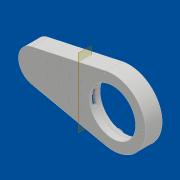
# Autodesk Inventor part: 101-bottom
Saved by Autodesk Inventor 2018 (Build 220112000, 112)
## iProperties
Created: 2019-11-07
Part Number: 101-bottom
Material: Generic
Document SubType Name: Modeling
Designer: Bunny320
Density: 1 g/cm^3
Appearance: Default
Author: Bunny320
Autodesk Inventor part; units mm, degrees
ref_plane "XZ Plane" through (0, 0, 0) normal (0, 1, 0) x (-1, 0, 0)
ref_plane "XY Plane" through (0, 0, 0) normal (0, 0, 1) x (1, 0, 0)
sketch "Sketch2" plane through (0, 0, 0) normal (0, 1, 0) x (-1, 0, 0)
  circle A0 centre (0, 0) radius 27.5
  circle A1 centre (-141.8, 0) radius 57.5
  line L0 (5.8181, -26.8775) -> (-129.635, -56.1984)
  line L1 (5.8181, 26.8775) -> (-129.635, 56.1984)
  dimension "d5" = 141.8
  dimension "d6" = 55
  dimension "d7" = 115
  constraints: 4 end point, 4 point on circle, 4 tangent, 2 centre point, 1 coincident, 1 horizontal alignment
  measures "d5" distance of A1.centre point (0, 0)
  measures "d6" diameter of A0
  measures "d7" diameter of A1
extrude "Extrusion2" add sketch "Sketch2" along normal blind 4
sketch "Sketch5" plane through (0, 4, 0) normal (0, 1, 0) x (1, 0, 0)
  arc A0 (129.635, -56.1984) -> (129.635, 56.1984) centre (141.8, 0) ccw projected
  circle A1 centre (141.8, 0) radius 45
  circle A2 centre (141.8, 0) radius 48
  point P0 (0, 0)
  dimension "d17" = 90
  dimension "d18" = 96
  constraints: 2 centre point, 2 coincident
  measures "d17" diameter of A1
  measures "d18" diameter of A2
extrude "Extrusion5" add sketch "Sketch5" along normal blind 18
sketch "Sketch6" plane through (141.8, 4, 0) normal (0, 1, 0) x (1, 0, 0)
  arc A0 (-12.165, -56.1984) -> (-12.165, 56.1984) centre (0, 0) ccw projected
  circle A1 centre (0, 0) radius 42
  point P0 (-141.8, 0)
  dimension "d21" = 84
  constraints: 1 centre point, 1 coincident
  measures "d21" diameter of A1
extrude "Extrusion6" cut sketch "Sketch6" against normal through all
sketch "Sketch9" plane through (0, 4, 0) normal (0, 1, 0) x (1, 0, 0)
  line L0 (-5.5, -9) -> (5.5, -9) construction
  line L1 (5.5, -9) -> (5.5, 9) construction
  line L2 (5.5, 9) -> (-5.5, 9) construction
  line L3 (-5.5, 9) -> (-5.5, -9) construction
  line L4 (-5.5, -9) -> (5.5, 9) construction
  line L5 (5.5, -9) -> (-5.5, 9) construction
  circle A0 centre (5.5, 9) radius 3
  circle A1 centre (-5.5, 9) radius 3
  circle A2 centre (-5.5, -9) radius 3
  circle A3 centre (5.5, -9) radius 3
  point P0 (0, 0)
  dimension "d33" = 11
  dimension "d34" = 18
  dimension "d35" = 6
  constraints: 12 end point, 4 centre point, 4 coincident, 3 equal radius, 2 midpoint, 2 parallel, 1 horizontal, 1 perpendicular
  measures "d33" distance of L1.end L2.end
  measures "d34" distance of L2.end L0.start
  measures "d35" diameter of A1
extrude "Extrusion7" add sketch "Sketch9" along normal blind 9.75
sketch "Sketch10" plane through (5.5, 13.75, -9) normal (0, 1, 0) x (1, 0, 0)
  circle A0 centre (-11, 0) radius 3 projected
  circle A1 centre (-11, -18) radius 3 projected
  circle A2 centre (0, -18) radius 3 projected
  circle A3 centre (0, 0) radius 3 projected
  point P0 (-5.5, -9)
  constraints: 4 coincident
hole "Hole2" at (-5.5, 13.75, -9) at (-5.5, 13.75, 9) at (5.5, 13.75, 9) at (5.5, 13.75, -9) direction (0, -1, 0) diameter 2.013 end through all thread size "M2.5x0.45" class "6H" standard "ISO Metric profile"
sketch "Sketch11" plane through (141.8, 4, 0) normal (0, 1, 0) x (1, 0, 0)
  circle A0 centre (0, 0) radius 42
  circle A1 centre (0, 0) radius 45.1248
  point P0 (-141.8, 0)
  constraints: 2 centre point, 1 coincident
extrude "Extrusion8" add sketch "Sketch11" along normal blind 8
ref_plane "Work Plane1" through (80, 0, 0) normal (1, 0, 0) x (0, 1, 0)
sketch "Sketch12" plane through (80, 0, 0) normal (1, 0, 0) x (0, 1, 0)
  line L0 (12, -15) -> (4, -15)
  line L1 (4, -15) -> (4, 15)
  line L2 (4, 15) -> (12, 15)
  line L3 (12, 15) -> (12, -15)
  line L4 (12, -15) -> (4, 15) construction
  line L5 (4, -15) -> (12, 15) construction
  line L6 (-2.4, 0) -> (14.4, 0) projected
  line L7 (4, -26.8775) -> (4, 26.8775) projected
  point P0 (0, 0)
  point P1 (8, 0)
  dimension "d48" = 8
  dimension "d49" = 30
  dimension "d50" = 0
  constraints: 12 end point, 2 midpoint, 2 parallel, 1 horizontal, 1 perpendicular, 1 point on line
  measures "d48" distance of L1.end L2.end
  measures "d49" distance of L2.end L0.start
  measures "d50" distance between parallel lines of L7 L1
extrude "Extrusion9" cut sketch "Sketch12" along normal blind 50
sketch "Sketch14" plane through (0, 0, 0) normal (0, 1, 0) x (-1, 0, 0)
  arc A0 (5.8181, -26.8775) -> (5.8181, 26.8775) centre (0, 0) ccw projected
  arc A1 (6.4528, -29.8096) -> (6.4528, 29.8096) centre (0, 0) ccw
  arc A2 (-129.635, 56.1984) -> (-129.635, -56.1984) centre (-141.8, 0) ccw projected
  arc A3 (-129.0003, 59.1305) -> (-129.0003, -59.1305) centre (-141.8, 0) ccw
  line L0 (6.4528, -29.8096) -> (-129.0003, -59.1305)
  line L1 (-129.0003, 59.1305) -> (6.4528, 29.8096)
  line L2 (-129.8465, -55.2211) -> (5.6065, -25.9001)
  arc A4 (5.6065, -25.9001) -> (5.6065, 25.9001) centre (0, 0) ccw
  line L3 (5.6065, 25.9001) -> (-129.8465, 55.2211)
  arc A5 (-129.8465, 55.2211) -> (-129.8465, -55.2211) centre (-141.8, 0) ccw
  dimension "d53" = 3
  dimension "d54" = 3
  dimension "d55" = 4
  constraints: 8 end point, 8 point on circle, 4 centre point, 4 tangent, 2 coincident, 3 other
  measures "d53" radial gap between concentric circles of A0 A1
  measures "d54" radial gap between concentric circles of A2 A3
  measures "d55" distance between parallel lines of L2 L0
extrude "Extrusion11" add sketch "Sketch14" along normal blind 30
sketch "Sketch15" plane through (0, 4, 0) normal (0, 1, 0) x (1, 0, 0)
  point P0 (0, 0)
  point P1 (25, 20)
  dimension "d60" = 25
  dimension "d61" = 20
  measures "d60" horizontal distance of point (0, 0) point (25, 20)
  measures "d61" vertical distance of point (25, 20) point (0, 0)
hole "Hole3" at (25, 4, -20) direction (0, -1, 0) diameter 2.459 end through all thread size "M3x0.5" class "6H" standard "ISO Metric profile"
pattern_linear "Rectangular Pattern1" count 4 spacing 20 along (1, 0, 0) count 3 spacing 20 along (0, 0, 1) of "Hole3"
sketch "Sketch16" plane through (-5.6065, 4, 25.9001) normal (0.2115656, 0, -0.9773638) x (-0.9773638, 0, -0.2115656)
  line L0 (0, 0) -> (-138.5902, 0) projected
  line L1 (0, 0) -> (-8, 0)
  line L2 (-8, 0) -> (-8, 26)
  line L3 (-8, 26) -> (0, 26)
  line L4 (0, 26) -> (0, 0)
  line L5 (-138.5902, 26) -> (0, 26) projected
  line L6 (-53, 0) -> (-61, 0)
  line L7 (-61, 0) -> (-61, 26)
  line L8 (-61, 26) -> (-53, 26)
  line L9 (-53, 26) -> (-53, 0)
  point P0 (0, -4)
  dimension "d75" = 8
  dimension "d78" = 8
  dimension "d79" = 45
  constraints: 16 end point, 4 parallel, 2 horizontal, 2 perpendicular, 2 point on line, 1 collinear
  measures "d75" distance of L2.end L3.end
  measures "d78" distance between parallel lines of L7 L9
  measures "d79" distance between parallel lines of L9 L2
extrude "Extrusion12" add sketch "Sketch16" along normal blind 4 contours L0 L2 L3 L4 | L0 L7 L5 L9
sketch "Sketch17" plane through (0, 30, 0) normal (0, 1, 0) x (1, 0, 0)
  line L0 (-4.7602, -21.9907) -> (3.0587, -23.6832) projected
  line L1 (3.0587, -23.6832) -> (-6.4327, -29.717)
  line L2 (-6.4327, -29.717) -> (-4.7401, -21.8975)
  line L3 (-4.7401, -21.8975) -> (1.366, -31.5027)
  line L4 (46.1938, -37.1131) -> (47.0401, -33.2037) projected
  line L5 (47.0401, -33.2037) -> (53.1865, -42.6225)
  line L6 (47.0401, -33.2037) -> (54.859, -34.8962) projected
  line L7 (54.859, -34.8962) -> (45.3474, -41.0231)
  point P0 (0, 0)
  point P1 (-1.687, -26.7001)
  point P2 (50.1032, -37.9597)
  constraints: 10 end point, 2 midpoint, 1 perpendicular, 1 point on line
hole "Hole4" at (-1.687, 30, 26.7001) at (50.1032, 30, 37.9597) direction (0, -1, 0) diameter 2.459 end through all thread size "M3x0.5" class "6H" standard "ISO Metric profile"
mirror "Mirror1" about plane through (0, 0, 0) normal (0, 0, 1) of "Extrusion12", "Hole4"
sketch "Sketch18" plane through (0, 4, 0) normal (0, 1, 0) x (1, 0, 0)
  line L0 (193.8, -4) -> (201.8, -4)
  line L1 (201.8, -4) -> (201.8, 4)
  line L2 (201.8, 4) -> (193.8, 4)
  line L3 (193.8, 4) -> (193.8, -4)
  line L4 (193.8, -4) -> (201.8, 4) construction
  line L5 (201.8, -4) -> (193.8, 4) construction
  arc A0 (102.5699, -15) -> (102.5699, 15) centre (141.8, 0) ccw projected
  arc A1 (129.8465, -55.2211) -> (129.8465, 55.2211) centre (141.8, 0) ccw projected
  line L6 (129.8465, -55.2211) -> (122.0276, -53.5285)
  line L7 (122.0276, -53.5285) -> (122.8739, -49.6191)
  line L8 (122.8739, -49.6191) -> (130.6928, -51.3116)
  line L9 (130.6928, -51.3116) -> (129.8465, -55.2211)
  line L10 (129.8465, 55.2211) -> (122.0276, 53.5285)
  line L11 (122.0276, 53.5285) -> (122.8739, 49.6191)
  line L12 (122.8739, 49.6191) -> (130.6928, 51.3116)
  line L13 (130.6928, 51.3116) -> (129.8465, 55.2211)
  line L14 (54.0127, 38.8056) -> (129.8465, 55.2211) projected
  point P0 (0, 0)
  point P1 (197.8, 0)
  dimension "d87" = 8
  dimension "d88" = 56
  dimension "d89" = 4
  dimension "d90" = 4
  dimension "d92" = 8
  dimension "d93" = 8
  constraints: 28 end point, 6 parallel, 4 perpendicular, 2 midpoint, 1 collinear, 1 horizontal, 1 horizontal alignment, 1 tangent
  measures "d87" distance between parallel lines of L0 L2
  measures "d88" distance of A0.centre point (197.8, 0)
  measures "d89" distance of L10.end L11.end
  measures "d90" distance of L6.end L7.end
  measures "d92" distance of L7.end L8.end
  measures "d93" distance of L11.end L12.end
extrude "Extrusion13" add sketch "Sketch18" along normal up to surface (26 mm away)
sketch "Sketch19" plane through (0, 30, 0) normal (0, 1, 0) x (1, 0, 0)
  line L0 (122.0276, -53.5285) -> (54.0127, -38.8056) projected
  line L1 (54.0127, 38.8056) -> (122.0276, 53.5285) projected
  line L2 (122.0276, 53.5285) -> (122.8739, 49.6191) projected
  line L3 (122.8739, -49.6191) -> (122.0276, -53.5285) projected
  circle A0 centre (141.8, 0) radius 48 projected
  point P0 (0, 0)
  point P1 (125.9371, 54.3748)
  point P2 (125.9371, -54.3748)
  point P3 (197.8, 0)
  dimension "d97" = 4
  dimension "d98" = 4
  dimension "d99" = 56
  constraints: 2 point on line, 1 horizontal alignment
  measures "d97" distance from line of L3 point (125.937, -54.375)
  measures "d98" distance from line of L2 point (125.937, 54.375)
  measures "d99" distance of A0.centre point (197.8, 0)
hole "Hole5" at (125.9371, 30, -54.3748) at (125.9371, 30, 54.3748) at (197.8, 30, 0) direction (0, -1, 0) diameter 2.459 end through all thread size "M3x0.5" class "6H" standard "ISO Metric profile"
sketch "Sketch20" plane through (2.2124, 4, -27.5927) normal (0.2115656, 0, 0.9773638) x (0.9773638, 0, -0.2115656)
  circle A0 centre (15, 12) radius 7.5
  line L0 (45, 0) -> (0, 0) projected
  line L1 (0, 26) -> (0, 0) projected
  point P0 (-8, -4)
  dimension "d107" = 12
  dimension "d108" = 15
  dimension "d109" = 15
  constraints: 1 centre point
  measures "d107" distance from line of L0 A0.centre
  measures "d108" diameter of A0
  measures "d109" distance from line of L1 A0.centre
extrude "Extrusion14" cut sketch "Sketch20" against normal through all
sketch "Sketch8" plane through (0, 4, 0) normal (0, 1, 0) x (1, 0, 0)
  line L0 (-5.5, 9) -> (5.5, 9)
  line L1 (5.5, 9) -> (5.5, -9)
  line L2 (5.5, -9) -> (-5.5, -9)
  line L3 (-5.5, -9) -> (-5.5, 9)
  line L4 (-5.5, 9) -> (5.5, -9) construction
  line L5 (5.5, 9) -> (-5.5, -9) construction
  point P0 (0, 0)
  dimension "d24" = 18
  dimension "d25" = 11
  constraints: 12 end point, 4 coincident, 2 midpoint, 2 parallel, 1 horizontal, 1 perpendicular
  measures "d24" distance of L2.end L0.start
  measures "d25" distance of L0.start L0.end
equation "\"d54\" = d53"
equation "\"d78\" = d75"
equation "\"d89\" = d90"
equation "\"d93\" = d92"
equation "\"d98\" = d97"
body "Solid2"
